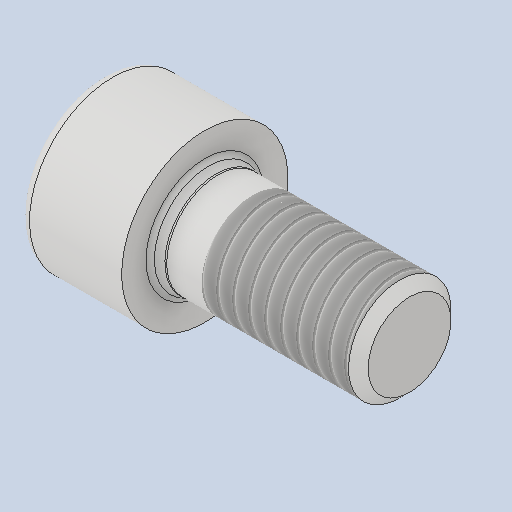
# Autodesk Inventor part: Robotunits IBS M8x16
Saved by Autodesk Inventor 2023 (Build 270158000, 158)
## iProperties
Created: 2023-08-22
Part Number: Robotunits IBS M8x16
Material: Generic
Catalog Web Link: www.cadenas.de
Description: IBS-Hexagon socket slotted head cap screw
Vendor: ROBOTUNITS
Document SubType Name: Modeling
Designer: psAdmin
Manufacturer: ROBOTUNITS
Mass: 1.68478 g
Surface Area: 10.6502 cm^2
Volume: 1.68478 cm^3
Density: 1 g/cm^3
Appearance: PSOLRGB-218-218-218
Category: PARTsolutions
Company: ROBOTUNITS
PSOL_IDENT_0: {$CADENAS_DATA/23d-libs/robotunits/pool_bauteile/schraube_ibs.prj},169 {VTYP=3D},{NB=Robotunits IBS
PSOL_IDENT_1: M8x16},{LINA=Robotunits IBS M8x16},{NN=IBS},{DATE=17.01.2023 14:45:04},{GEOMDATE=01.06.2004},{VERSIO
PSOL_IDENT_2: N=},{LINEID=800},{WBVAR=},{WBNUMERIC=}  {NB=Robotunits IBS M8x16},{LINA=Robotunits IBS M8x16},{KT=X}
PSOL_IDENT_3: ,{GEW=M8},{D=8.000},{D3=6.466},{P=1.250},{L=16.000},{B=16.000},{S=6.000},{DK=13.000},{K=8.000},{DA=9
PSOL_IDENT_4: .200},{DW=12.330},{DS=8.000},{A=1.020},{R=0.400},{T=4.000},{V=0.800},{E=6.860},{W=3.000},{LG=3.750},
PSOL_IDENT_5: {NENN=M8x16},{FORM=1.000},{KOPFFORM=Zylinderkopf}
NB: Robotunits IBS M8x16
NN: IBS
NT: Hexagon socket slotted head cap screw
NBSYN: Robotunits IBS $NENN.
LINA: Robotunits IBS M8x16
CATALOG: Robotunits
ROWDESC: M8x16
D: 8
D3: 6.466
P: 1.25
L: 16
B: 16
S: 6
DK: 13
K: 8
DA: 9.2
DW: 12.33
DS: 8
A: 1.02
R: 0.4
T: 4
V: 0.8
E: 6.86
W: 3
LG: 3.75
FORM: 1
SUPPLIER: ROBOTUNITS
ARTICLENO: Robotunits IBS M8x16
BOMINFO: Robotunits IBS M8x16
CREATOR: CADENAS GmbH
Title: Robotunits IBS M8x16
Author: Cadenas PARTsolutions
Comments: Hexagon socket slotted head cap screw
Autodesk Inventor part; units mm, degrees
sketch "Skizze_2" plane through (0, 0, 0) normal (0, 0, 1) x (1, 0, 0)
  line L0 (19, 0) -> (-11, 0)
  line L1 (-1.2679, 0) -> (-3, 3)
  line L2 (-3, 3) -> (-7.57, 3)
  line L3 (-7.57, 3) -> (-8, 3.43)
  line L4 (-8, 3.43) -> (-8, 5.7)
  arc A0 (-7.2, 6.5) -> (-8, 5.7) centre (-7.2, 5.7) ccw
  line L5 (-7.2, 6.5) -> (0, 6.5)
  line L6 (0, 6.5) -> (0, 4.6)
  arc A1 (0, 4.6) -> (0.2772, 4.2193) centre (0.4, 4.6) ccw
  line L7 (0.2772, 4.2193) -> (0.8972, 4.0193)
  arc A2 (0.8972, 4.0193) -> (1.02, 4) centre (1.02, 4.4) ccw
  line L8 (1.02, 4) -> (15.233, 4)
  line L9 (15.233, 4) -> (16, 3.233)
  line L10 (16, 3.233) -> (16, 0)
  line L11 (16, 0) -> (-1.2679, 0)
  constraints: 24 end point, 6 point on circle, 3 centre point
revolve "Revolution1" add sketch "Skizze_2" angle 360 about axis through (19, 0, 0) along (1, 0, 0)
thread "Thread1" size "M8x1.25" class "6g" standard "ISO Metric profile" length 11.483
sketch "Skizze_1" plane through (-3, 0, 0) normal (1, 0, 0) x (0, 0, -1)
  line L0 (-3, -1.7321) -> (0, -3.4641)
  line L1 (0, -3.4641) -> (3, -1.7321)
  line L2 (3, -1.7321) -> (3, 1.7321)
  line L3 (3, 1.7321) -> (0, 3.4641)
  line L4 (0, 3.4641) -> (-3, 1.7321)
  line L5 (-3, 1.7321) -> (-3, -1.7321)
  constraints: 12 end point
extrude "Extrusion1" cut sketch "Skizze_1" against normal blind 8
ref_plane "IP1_XY" through (0, 0, 0) normal (1, 0, 0) x (0, 0, -1)
ref_plane "IP1_YZ" through (0, 0, 0) normal (0, 0, -1) x (0, 1, 0)
ref_plane "IP1_ZX" through (0, 0, 0) normal (0, 1, 0) x (1, 0, 0)
ref_plane "IP2_XY" through (-8, 0, 0) normal (1, 0, 0) x (0, 0, -1)
ref_plane "IP2_YZ" through (-8, 0, 0) normal (0, 0, -1) x (0, 1, 0)
ref_plane "IP2_ZX" through (-8, 0, 0) normal (0, 1, 0) x (1, 0, 0)
ref_plane "IP3_XY" through (16, 0, 0) normal (1, 0, 0) x (0, 0, -1)
ref_plane "IP3_YZ" through (16, 0, 0) normal (0, 0, -1) x (0, 1, 0)
ref_plane "IP3_ZX" through (16, 0, 0) normal (0, 1, 0) x (1, 0, 0)
ref_plane "P_GUS_1000_XY" through (11.5, 0, 0) normal (1, 0, 0) x (0, 0, -1)
ref_plane "P_GUS_1000_YZ" through (11.5, 0, 0) normal (0, 0, -1) x (0, 1, 0)
ref_plane "P_GUS_1000_ZX" through (11.5, 0, 0) normal (0, 1, 0) x (1, 0, 0)
body "Solid1"
